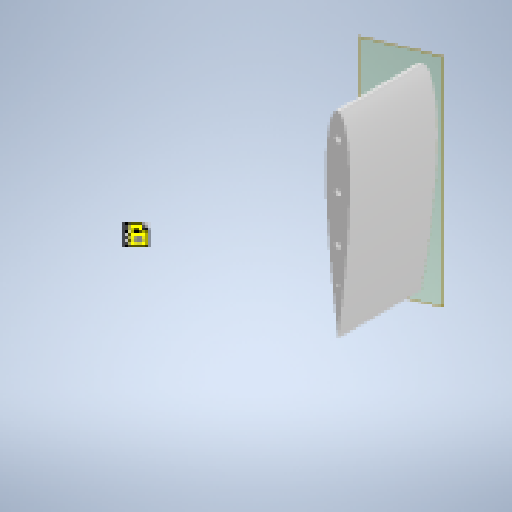
# Autodesk Inventor part: Part1
Saved by Autodesk Inventor 2025.2 (Build 292293000, 293)
## iProperties
Created: 2025-02-19
Part Number: Part1
Material: Generic
Document SubType Name: Modeling
Designer: georg
Density: 1 g/cm^3
Appearance: Default
Author: georg
Autodesk Inventor part; units mm, degrees
ref_plane "Work Plane1" through (0, 0, 0) normal (0, 1, 0) x (0, 0, 1)
ref_plane "Work Plane5" through (0, 0, 0) normal (1, 0, 0) x (0, 0, -1)
sketch "Sketch15" plane through (0, 0, 0) normal (0, 0, 1) x (1, 0, 0)
  spline S0 degree 5 poles (0, -203.2) (0.0023, -203.2) (0.0066, -203.1673) (0.016, -203.012) (0.0464, -202.9995) (0.0761, -202.5642) (0.1335, -202.3714) (0.1917, -201.8117) (0.2746, -201.3405) (0.3648, -200.6481) (0.4721, -199.9314) (0.5911, -199.0751) (0.7234, -198.1458) (0.8688, -197.1087) (1.0256, -195.984) (1.1945, -194.7625) (1.3748, -193.4512) (1.5657, -192.0477) (1.767, -190.5558) (1.9786, -188.9759) (2.1986, -187.3097) (2.4282, -185.5589) (2.6657, -183.7252) (2.9115, -181.8108) (3.1632, -179.8167) (3.4229, -177.7459) (3.6879, -175.5995) (3.9581, -173.3803) (4.2337, -171.0905) (4.5134, -168.7317) (4.7966, -166.3068) (5.0834, -163.8182) (5.3725, -161.2679) (5.6631, -158.659) (5.956, -155.9934) (6.2488, -153.2746) (6.5425, -150.5045) (6.8348, -147.6861) (7.127, -144.8226) (7.4174, -141.916) (7.705, -138.9697) (7.9903, -135.9869) (8.2715, -132.9695) (8.549, -129.922) (8.8215, -126.8457) (9.0881, -123.745) (9.3491, -120.6224) (9.6026, -117.4806) (9.8495, -114.3238) (10.0866, -111.1538) (10.3164, -107.9748) (10.5349, -104.7893) (10.7445, -101.6008) (10.942, -98.4123) (11.1277, -95.2267) (11.3009, -92.0477) (11.4615, -88.8777) (11.6069, -85.7208) (11.739, -82.5791) (11.8548, -79.4563) (11.9554, -76.3556) (12.039, -73.2792) (12.1057, -70.2316) (12.1549, -67.2141) (12.1854, -64.2311) (12.198, -61.2847) (12.1911, -58.378) (12.1652, -55.5142) (12.1197, -52.6956) (12.0539, -49.9253) (11.9681, -47.2063) (11.8622, -44.5404) (11.7355, -41.9312) (11.589, -39.3806) (11.4216, -36.8917) (11.2342, -34.4665) (11.0264, -32.1073) (10.7996, -29.817) (10.5524, -27.5973) (10.2861, -25.4503) (10.0015, -23.3788) (9.698, -21.3841) (9.3765, -19.469) (9.0379, -17.6343) (8.682, -15.8826) (8.3103, -14.2152) (7.9227, -12.634) (7.5202, -11.1404) (7.103, -9.7353) (6.6725, -8.4212) (6.2284, -7.198) (5.7722, -6.0677) (5.3036, -5.0307) (4.8237, -4.0882) (4.3332, -3.2402) (3.831, -2.4886) (3.3186, -1.832) (2.7948, -1.2726) (2.2592, -0.8103) (1.7116, -0.4465) (1.151, -0.1846) (0.5803, -0.0264) (0, 0.026) (-0.5803, -0.0264) (-1.151, -0.1846) (-1.7116, -0.4465) (-2.2592, -0.8103) (-2.7948, -1.2726) (-3.3186, -1.832) (-3.831, -2.4886) (-4.3332, -3.2402) (-4.8237, -4.0882) (-5.3036, -5.0307) (-5.7722, -6.0677) (-6.2284, -7.198) (-6.6725, -8.4212) (-7.103, -9.7353) (-7.5202, -11.1404) (-7.9227, -12.634) (-8.3103, -14.2152) (-8.682, -15.8826) (-9.0379, -17.6343) (-9.3765, -19.469) (-9.698, -21.3841) (-10.0015, -23.3788) (-10.2861, -25.4503) (-10.5524, -27.5973) (-10.7996, -29.817) (-11.0264, -32.1073) (-11.2342, -34.4665) (-11.4216, -36.8917) (-11.589, -39.3806) (-11.7355, -41.9312) (-11.8622, -44.5404) (-11.9681, -47.2063) (-12.0539, -49.9253) (-12.1197, -52.6956) (-12.1652, -55.5142) (-12.1911, -58.378) (-12.198, -61.2847) (-12.1854, -64.2311) (-12.1549, -67.2141) (-12.1057, -70.2316) (-12.039, -73.2792) (-11.9554, -76.3556) (-11.8548, -79.4563) (-11.739, -82.5791) (-11.6069, -85.7208) (-11.4615, -88.8777) (-11.3009, -92.0477) (-11.1277, -95.2267) (-10.942, -98.4123) (-10.7445, -101.6008) (-10.5349, -104.7893) (-10.3164, -107.9748) (-10.0866, -111.1538) (-9.8495, -114.3238) (-9.6026, -117.4806) (-9.3491, -120.6224) (-9.0881, -123.745) (-8.8215, -126.8457) (-8.549, -129.922) (-8.2715, -132.9695) (-7.9903, -135.9869) (-7.705, -138.9697) (-7.4174, -141.916) (-7.127, -144.8226) (-6.8348, -147.6861) (-6.5425, -150.5045) (-6.2488, -153.2746) (-5.956, -155.9934) (-5.6631, -158.659) (-5.3725, -161.2679) (-5.0834, -163.8182) (-4.7966, -166.3068) (-4.5134, -168.7317) (-4.2337, -171.0905) (-3.9581, -173.3803) (-3.6879, -175.5995) (-3.4229, -177.7459) (-3.1632, -179.8167) (-2.9115, -181.8108) (-2.6657, -183.7252) (-2.4282, -185.5589) (-2.1986, -187.3097) (-1.9786, -188.9759) (-1.767, -190.5558) (-1.5657, -192.0477) (-1.3748, -193.4512) (-1.1945, -194.7625) (-1.0256, -195.984) (-0.8688, -197.1087) (-0.7234, -198.1458) (-0.5911, -199.0751) (-0.4721, -199.9314) (-0.3648, -200.6481) (-0.2746, -201.3405) (-0.1917, -201.8117) (-0.1335, -202.3714) (-0.0761, -202.5642) (-0.0464, -202.9995) (-0.016, -203.012) (-0.0066, -203.1673) (-0.0023, -203.2) (0, -203.2) knots 0 0 0 0 0 0 0.00141 0.002644 0.004363 0.006456 0.008851 0.011509 0.014402 0.017511 0.020819 0.024314 0.027984 0.031819 0.03581 0.039949 0.044229 0.048644 0.053187 0.057852 0.062634 0.067528 0.072529 0.077632 0.082832 0.088126 0.093509 0.098976 0.104525 0.11015 0.115849 0.121616 0.12745 0.133346 0.1393 0.14531 0.15137 0.15748 0.163633 0.169829 0.176062 0.18233 0.188629 0.194957 0.201309 0.207683 0.214076 0.220484 0.226904 0.233333 0.239767 0.246204 0.25264 0.259072 0.265497 0.271912 0.278314 0.284699 0.291064 0.297407 0.303723 0.310011 0.316266 0.322485 0.328666 0.334804 0.340898 0.346943 0.352937 0.358876 0.364757 0.370576 0.376331 0.382017 0.387632 0.393172 0.398634 0.404014 0.409309 0.414515 0.419627 0.424644 0.42956 0.434371 0.439075 0.443667 0.448142 0.452498 0.456729 0.460831 0.464802 0.468638 0.472335 0.475892 0.479309 0.482586 0.485731 0.488751 0.491664 0.494492 0.497262 0.5 0.502738 0.505508 0.508336 0.511249 0.514269 0.517414 0.520691 0.524108 0.527665 0.531362 0.535198 0.539169 0.543271 0.547502 0.551858 0.556333 0.560925 0.565629 0.57044 0.575356 0.580373 0.585485 0.590691 0.595986 0.601366 0.606828 0.612368 0.617983 0.623669 0.629424 0.635243 0.641124 0.647063 0.653057 0.659102 0.665196 0.671334 0.677515 0.683734 0.689989 0.696277 0.702593 0.708936 0.715301 0.721686 0.728088 0.734503 0.740928 0.74736 0.753796 0.760233 0.766667 0.773096 0.779516 0.785924 0.792317 0.798691 0.805043 0.811371 0.81767 0.823938 0.830171 0.836367 0.84252 0.84863 0.85469 0.8607 0.866654 0.87255 0.878384 0.884151 0.88985 0.895475 0.901024 0.906491 0.911874 0.917168 0.922368 0.927471 0.932472 0.937366 0.942148 0.946813 0.951356 0.955771 0.960051 0.96419 0.968181 0.972016 0.975686 0.979181 0.982489 0.985598 0.988491 0.991149 0.993544 0.995637 0.997356 0.99859 1 1 1 1 1 1
  point P0 (0, 0)
  point P1 (0.0291, -202.9994)
  point P2 (0.0654, -202.7491)
  point P3 (0.1162, -202.3988)
  point P4 (0.1811, -201.9491)
  point P5 (0.2601, -201.4005)
  point P6 (0.353, -200.7531)
  point P7 (0.4592, -200.0081)
  point P8 (0.5789, -199.1659)
  point P9 (0.7114, -198.2273)
  point P10 (0.8567, -197.1934)
  point P11 (1.014, -196.0652)
  point P12 (1.183, -194.8438)
  point P13 (1.3635, -193.5305)
  point P14 (1.5547, -192.1262)
  point P15 (1.7563, -190.6327)
  point P16 (1.9678, -189.0514)
  point P17 (2.1885, -187.3837)
  point P18 (2.4181, -185.6313)
  point P19 (2.656, -183.796)
  point P20 (2.9017, -181.8798)
  point P21 (3.1543, -179.8842)
  point P22 (3.4138, -177.8114)
  point P23 (3.6791, -175.6631)
  point P24 (3.9498, -173.442)
  point P25 (4.2255, -171.1501)
  point P26 (4.5056, -168.7893)
  point P27 (4.7892, -166.3623)
  point P28 (5.0761, -163.8715)
  point P29 (5.3655, -161.3191)
  point P30 (5.6567, -158.7077)
  point P31 (5.9495, -156.0399)
  point P32 (6.2429, -153.3187)
  point P33 (6.5365, -150.5462)
  point P34 (6.8296, -147.7254)
  point P35 (7.1218, -144.8592)
  point P36 (7.4123, -141.9502)
  point P37 (7.7005, -139.0014)
  point P38 (7.9858, -136.0158)
  point P39 (8.2674, -132.996)
  point P40 (8.545, -129.9456)
  point P41 (8.8177, -126.8669)
  point P42 (9.0847, -123.7634)
  point P43 (9.3456, -120.638)
  point P44 (9.5996, -117.4937)
  point P45 (9.8461, -114.3339)
  point P46 (10.084, -111.1614)
  point P47 (10.3132, -107.9795)
  point P48 (10.5325, -104.7913)
  point P49 (10.7416, -101.6)
  point P50 (10.9393, -98.4087)
  point P51 (11.125, -95.2205)
  point P52 (11.2983, -92.0386)
  point P53 (11.4584, -88.8661)
  point P54 (11.6043, -85.7063)
  point P55 (11.7358, -82.562)
  point P56 (11.8518, -79.4366)
  point P57 (11.952, -76.3331)
  point P58 (12.0355, -73.2544)
  point P59 (12.102, -70.204)
  point P60 (12.1508, -67.1842)
  point P61 (12.1812, -64.1986)
  point P62 (12.1932, -61.2498)
  point P63 (12.1861, -58.3408)
  point P64 (12.1597, -55.4746)
  point P65 (12.1136, -52.6538)
  point P66 (12.0473, -49.8813)
  point P67 (11.961, -47.1601)
  point P68 (11.8543, -44.4923)
  point P69 (11.7271, -41.8809)
  point P70 (11.5796, -39.3285)
  point P71 (11.4115, -36.8377)
  point P72 (11.2231, -34.4107)
  point P73 (11.0147, -32.0499)
  point P74 (10.7865, -29.758)
  point P75 (10.5384, -27.5369)
  point P76 (10.2709, -25.3886)
  point P77 (9.9848, -23.3158)
  point P78 (9.68, -21.3202)
  point P79 (9.3572, -19.404)
  point P80 (9.0168, -17.5687)
  point P81 (8.6594, -15.8163)
  point P82 (8.2857, -14.1486)
  point P83 (7.8961, -12.5673)
  point P84 (7.4914, -11.0738)
  point P85 (7.072, -9.6695)
  point P86 (6.6387, -8.3562)
  point P87 (6.1921, -7.1348)
  point P88 (5.7329, -6.0066)
  point P89 (5.2615, -4.9727)
  point P90 (4.7787, -4.0341)
  point P91 (4.2851, -3.1919)
  point P92 (3.7809, -2.4469)
  point P93 (3.267, -1.7995)
  point P94 (2.7438, -1.2509)
  point P95 (2.2116, -0.8012)
  point P96 (1.6709, -0.4509)
  point P97 (1.1219, -0.2006)
  point P98 (0.5647, -0.0502)
  point P99 (0, 0)
  point P100 (-0.5647, -0.0502)
  point P101 (-1.1219, -0.2006)
  point P102 (-1.6709, -0.4509)
  point P103 (-2.2116, -0.8012)
  point P104 (-2.7438, -1.2509)
  point P105 (-3.267, -1.7995)
  point P106 (-3.7809, -2.4469)
  point P107 (-4.2851, -3.1919)
  point P108 (-4.7787, -4.0341)
  point P109 (-5.2615, -4.9727)
  point P110 (-5.7329, -6.0066)
  point P111 (-6.1921, -7.1348)
  point P112 (-6.6387, -8.3562)
  point P113 (-7.072, -9.6695)
  point P114 (-7.4914, -11.0738)
  point P115 (-7.8961, -12.5673)
  point P116 (-8.2857, -14.1486)
  point P117 (-8.6594, -15.8163)
  point P118 (-9.0168, -17.5687)
  point P119 (-9.3572, -19.404)
  point P120 (-9.68, -21.3202)
  point P121 (-9.9848, -23.3158)
  point P122 (-10.2709, -25.3886)
  point P123 (-10.5384, -27.5369)
  point P124 (-10.7865, -29.758)
  point P125 (-11.0147, -32.0499)
  point P126 (-11.2231, -34.4107)
  point P127 (-11.4115, -36.8377)
  point P128 (-11.5796, -39.3285)
  point P129 (-11.7271, -41.8809)
  point P130 (-11.8543, -44.4923)
  point P131 (-11.961, -47.1601)
  point P132 (-12.0473, -49.8813)
  point P133 (-12.1136, -52.6538)
  point P134 (-12.1597, -55.4746)
  point P135 (-12.1861, -58.3408)
  point P136 (-12.1932, -61.2498)
  point P137 (-12.1812, -64.1986)
  point P138 (-12.1508, -67.1842)
  point P139 (-12.102, -70.204)
  point P140 (-12.0355, -73.2544)
  point P141 (-11.952, -76.3331)
  point P142 (-11.8518, -79.4366)
  point P143 (-11.7358, -82.562)
  point P144 (-11.6043, -85.7063)
  point P145 (-11.4584, -88.8661)
  point P146 (-11.2983, -92.0386)
  point P147 (-11.125, -95.2205)
  point P148 (-10.9393, -98.4087)
  point P149 (-10.7416, -101.6)
  point P150 (-10.5325, -104.7913)
  point P151 (-10.3132, -107.9795)
  point P152 (-10.084, -111.1614)
  point P153 (-9.8461, -114.3339)
  point P154 (-9.5996, -117.4937)
  point P155 (-9.3456, -120.638)
  point P156 (-9.0847, -123.7634)
  point P157 (-8.8177, -126.8669)
  point P158 (-8.545, -129.9456)
  point P159 (-8.2674, -132.996)
  point P160 (-7.9858, -136.0158)
  point P161 (-7.7005, -139.0014)
  point P162 (-7.4123, -141.9502)
  point P163 (-7.1218, -144.8592)
  point P164 (-6.8296, -147.7254)
  point P165 (-6.5365, -150.5462)
  point P166 (-6.2429, -153.3187)
  point P167 (-5.9495, -156.0399)
  point P168 (-5.6567, -158.7077)
  point P169 (-5.3655, -161.3191)
  point P170 (-5.0761, -163.8715)
  point P171 (-4.7892, -166.3623)
  point P172 (-4.5056, -168.7893)
  point P173 (-4.2255, -171.1501)
  point P174 (-3.9498, -173.442)
  point P175 (-3.6791, -175.6631)
  point P176 (-3.4138, -177.8114)
  point P177 (-3.1543, -179.8842)
  point P178 (-2.9017, -181.8798)
  point P179 (-2.656, -183.796)
  point P180 (-2.4181, -185.6313)
  point P181 (-2.1885, -187.3837)
  point P182 (-1.9678, -189.0514)
  point P183 (-1.7563, -190.6327)
  point P184 (-1.5547, -192.1262)
  point P185 (-1.3635, -193.5305)
  point P186 (-1.183, -194.8438)
  point P187 (-1.014, -196.0652)
  point P188 (-0.8567, -197.1934)
  point P189 (-0.7114, -198.2273)
  point P190 (-0.5789, -199.1659)
  point P191 (-0.4592, -200.0081)
  point P192 (-0.353, -200.7531)
  point P193 (-0.2601, -201.4005)
  point P194 (-0.1811, -201.9491)
  point P195 (-0.1162, -202.3988)
  point P196 (-0.0654, -202.7491)
  point P197 (-0.0291, -202.9994)
  point P198 (-0.0073, -203.1498)
  constraints: 1 coincident, 200 other
extrude "Extrusion11" add sketch "Sketch15" along normal blind 91.938
sketch "Sketch21" plane through (0, 0, 0) normal (0, 1, 0) x (-1, 0, 0)
  line L0 (-14.7334, 0) -> (14.7334, 12.2055)
  line L1 (14.7334, 0) -> (-14.7334, 0)
  line L2 (14.7334, 0) -> (14.7334, 12.2055)
  line L3 (14.7334, 12.2055) -> (14.7334, 0)
  line L4 (-14.7334, 0) -> (14.7334, 0)
  point P0 (0, 0)
  point P1 (0, 0)
  point P2 (0, 0)
  dimension "d57" = 22.5
  constraints: 10 end point, 1 collinear, 1 point on line, 1 vertical
  measures "d57" angle of L0 L1
extrude "Extrusion14" cut sketch "Sketch21" along normal mid plane 508
sketch "Sketch22" plane through (0, 0, 91.938) normal (0, 0, 1) x (1, 0, 0)
  circle A0 centre (0, -156.3428) radius 1.5875
  circle A1 centre (0, -156.3428) radius 1.5875
  point P0 (0, 0)
  dimension "d58" = 3.175
  constraints: 2 centre point, 1 coincident, 1 vertical alignment, 2 other
  measures "d58" diameter of A0
extrude "Extrusion15" cut sketch "Sketch22" against normal blind 10
sketch "Sketch23" plane through (0, 0, 91.938) normal (0, 0, 1) x (1, 0, 0)
  circle A0 centre (0, -25.4) radius 3.175
  circle A1 centre (0, -120.26) radius 3.175
  circle A2 centre (0, -72.8255) radius 3.175
  point P0 (0, -203.2)
  dimension "d92" = 6.35
  dimension "d93" = 6.35
  dimension "d94" = 6.35
  dimension "d96" = 47.4345
  dimension "d97" = 47.4255
  constraints: 3 centre point
  measures "d92" diameter of A0
  measures "d93" diameter of A1
  measures "d94" diameter of A2
  measures "d96" distance of A1.centre A2.centre
  measures "d97" distance of A2.centre A0.centre
extrude "Extrusion16" cut sketch "Sketch23" against normal blind 25.4
ref_plane "Work Plane9" through (0, -203.2, 49.0204) normal (0, 0, 1) x (1, 0, 0)
ref_plane "Work Plane10" through (0, -203.2, 6.1028) normal (-0.3826834, 0, -0.9238795) x (-0.9238795, 0, 0.3826834)
sketch "Sketch28" plane through (0, -203.2, 6.1028) normal (-0.3826834, 0, -0.9238795) x (-0.9238795, 0, 0.3826834)
  circle A0 centre (0, 177.8) radius 3.175
  circle A1 centre (0, 82.94) radius 3.175
  circle A2 centre (0, 130.3745) radius 3.175
  point P0 (0, 0)
  dimension "d98" = 6.35
  dimension "d99" = 6.35
  dimension "d100" = 6.35
  dimension "d101" = 47.4345
  dimension "d102" = 47.4255
  constraints: 3 centre point
  measures "d98" diameter of A0
  measures "d99" diameter of A1
  measures "d100" diameter of A2
  measures "d101" distance of A1.centre A2.centre
  measures "d102" distance of A2.centre A0.centre
extrude "Extrusion17" cut sketch "Sketch28" against normal blind 12.7
body "Solid2"
